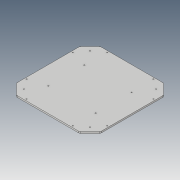
# Autodesk Inventor part: bottomPlate
Saved by Autodesk Inventor 2018 (Build 220112000, 112)
## iProperties
Created: 2019-11-22
Part Number: bottomPlate
Material: Generic
Document SubType Name: Modeling
Designer: anirudh
Density: 1 g/cm^3
Appearance: Default
Author: anirudh
Autodesk Inventor part; units mm, degrees
ref_plane "YZ Plane" through (0, 0, 0) normal (1, 0, 0) x (0, 1, 0)
ref_plane "XZ Plane" through (0, 0, 0) normal (0, 1, 0) x (-1, 0, 0)
ref_plane "XY Plane" through (0, 0, 0) normal (0, 0, 1) x (1, 0, 0)
sketch "Sketch1" plane through (0, 0, 0) normal (0, 1, 0) x (-1, 0, 0)
  line L0 (304.8, -38.1) -> (304.8, -266.7)
  line L1 (266.7, -304.8) -> (38.1, -304.8)
  line L2 (0, -266.7) -> (0, -38.1)
  line L3 (0, -38.1) -> (38.1, 0)
  line L4 (38.1, 0) -> (266.7, 0)
  line L5 (266.7, 0) -> (304.8, -38.1)
  line L6 (0, -266.7) -> (38.1, -304.8)
  line L7 (266.7, -304.8) -> (304.8, -266.7)
  circle A0 centre (238.125, -87.3125) radius 1.85
  circle A1 centre (66.675, -87.3125) radius 1.85
  circle A2 centre (66.675, -217.4875) radius 1.85
  circle A3 centre (238.125, -217.4875) radius 1.85
  point P0 (0, 0)
  dimension "d10" = 3.7
  dimension "d11" = 3.7
  dimension "d12" = 3.7
  dimension "d13" = 3.7
  constraints: 16 end point, 4 centre point, 1 parallel, 1 perpendicular
  measures "d10" diameter of A0
  measures "d11" diameter of A1
  measures "d12" diameter of A2
  measures "d13" diameter of A3
extrude "Extrusion1" add sketch "Sketch1" along normal blind 5.588
fillet "Fillet1" radius 6.35 8 edges at (-38.1, 2.794, 0) (0, 2.794, -38.1) (0, 2.794, -266.7) (-38.1, 2.794, -304.8) (-266.7, 2.794, 0) (-304.8, 2.794, -38.1) (-304.8, 2.794, -266.7) (-266.7, 2.794, -304.8)
sketch "Sketch2" plane through (0, 5.588, 0) normal (0, 1, 0) x (1, 0, 0)
  circle A0 centre (-68.5771, 6.3529) radius 1.85
  circle A1 centre (-68.5771, 6.3529) radius 1.85
  circle A2 centre (-32.5204, 32.5204) radius 1.85
  circle A3 centre (-6.3529, 68.5771) radius 1.85
  circle A4 centre (-6.3529, 68.5771) radius 1.85
  line L0 (-264.0697, 0) -> (-40.7303, 0) projected
  line L1 (-264.0697, 304.8) -> (-40.7303, 304.8) projected
  line L2 (-304.8, 264.0697) -> (-304.8, 40.7303) projected
  line L3 (0, 264.0697) -> (0, 40.7303) projected
  circle A5 centre (-68.5771, 298.4471) radius 1.85
  circle A6 centre (-68.5771, 298.4471) radius 1.85
  circle A7 centre (-32.5204, 272.2796) radius 1.85
  circle A8 centre (-6.3529, 236.2229) radius 1.85
  circle A9 centre (-6.3529, 236.2229) radius 1.85
  circle A10 centre (-236.2229, 6.3529) radius 1.85
  circle A11 centre (-236.2229, 6.3529) radius 1.85
  circle A12 centre (-272.2796, 32.5204) radius 1.85
  circle A13 centre (-298.4471, 68.5771) radius 1.85
  circle A14 centre (-298.4471, 68.5771) radius 1.85
  circle A15 centre (-236.2229, 298.4471) radius 1.85
  circle A16 centre (-236.2229, 298.4471) radius 1.85
  circle A17 centre (-272.2796, 272.2796) radius 1.85
  circle A18 centre (-298.4471, 236.2229) radius 1.85
  circle A19 centre (-298.4471, 236.2229) radius 1.85
  point P0 (-36.2401, 1.8599)
  constraints: 20 centre point, 8 coincident
extrude "Extrusion2" cut sketch "Sketch2" against normal blind 16.7005
body "Solid1"
